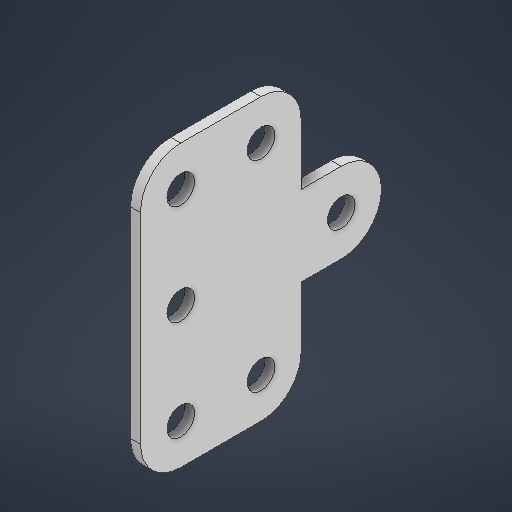
# Autodesk Inventor part: polygusset
Saved by Autodesk Inventor 2025.2 (Build 292293000, 293)
## iProperties
Created: 2025-04-08
Part Number: polygusset
Material: Generic
Document SubType Name: Modeling
Designer: roejo
Density: 1 g/cm^3
Appearance: Default
Author: roejo
Autodesk Inventor part; units mm, degrees
ref_plane "YZ Plane" through (0, 0, 0) normal (1, 0, 0) x (0, 1, 0)
ref_plane "XZ Plane" through (0, 0, 0) normal (0, 1, 0) x (-1, 0, 0)
ref_plane "XY Plane" through (0, 0, 0) normal (0, 0, 1) x (1, 0, 0)
sketch "Sketch1" plane through (0, 0, 0) normal (1, 0, 0) x (0, 1, 0)
  arc A0 (-6.35, -25.4) -> (6.35, -25.4) centre (0, -25.4) ccw
  line L0 (-6.35, -19.05) -> (-15.875, -19.05)
  circle A1 centre (-15.875, -12.7) radius 2.1844
  arc A2 (-22.225, -12.7) -> (-15.875, -19.05) centre (-15.875, -12.7) ccw
  line L1 (-6.35, -25.4) -> (-6.35, -19.05)
  circle A3 centre (15.875, -12.7) radius 2.1844
  arc A4 (15.875, -19.05) -> (22.225, -12.7) centre (15.875, -12.7) ccw
  line L2 (15.875, -19.05) -> (6.35, -19.05)
  line L3 (6.35, -19.05) -> (6.35, -25.4)
  circle A5 centre (0, 0) radius 2.1844
  circle A6 centre (0, -25.4) radius 2.1844
  line L4 (0, 6.35) -> (6.35, 6.35)
  line L5 (0, 6.35) -> (-6.35, 6.35)
  line L6 (-15.875, 6.35) -> (15.875, 6.35)
  line L7 (22.225, 0) -> (22.225, -12.7)
  line L8 (-6.35, 6.35) -> (-15.875, 6.35)
  line L9 (-22.225, 0) -> (-22.225, -12.7)
  circle A7 centre (15.875, 0) radius 2.1844
  circle A8 centre (-15.875, 0) radius 2.1844
  arc A9 (-15.875, 6.35) -> (-22.225, 0) centre (-15.875, 0) ccw
  arc A10 (22.225, 0) -> (15.875, 6.35) centre (15.875, 0) ccw
  dimension "d22" = 4.3688
  dimension "d23" = 4.3688
  dimension "d25" = 4.3688
  dimension "d27" = 4.3688
  dimension "d28" = 6.35
  constraints: 20 end point, 11 centre point, 10 point on circle, 7 tangent, 4 horizontal, 3 coincident, 2 perpendicular, 1 equal radius, 1 point on line
  measures "d22" diameter of A5
  measures "d23" diameter of A6
  measures "d25" diameter of A7
  measures "d27" diameter of A8
  measures "d28" radius of A9
extrude "Extrusion1" add sketch "Sketch1" along normal blind 1.5875
body "Solid1"
